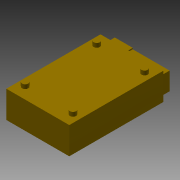
# Autodesk Inventor part: Vilros Pi Case
Saved by Autodesk Inventor 2015 SP1 (Build 190203100, 203)
## iProperties
Created: 2015-03-20
Part Number: Vilros Pi Case
Material: Generic
Document SubType Name: Modeling
Designer: steele
Density: 1 g/cm^3
Appearance: Gold
Author: steele
Autodesk Inventor part; units mm, degrees
ref_plane "YZ Plane" through (0, 0, 0) normal (1, 0, 0) x (0, 1, 0)
ref_plane "XZ Plane" through (0, 0, 0) normal (0, 1, 0) x (-1, 0, 0)
ref_plane "XY Plane" through (0, 0, 0) normal (0, 0, 1) x (1, 0, 0)
sketch "Sketch1" plane through (0, 0, 0) normal (0, 0, 1) x (1, 0, 0)
  line L0 (-30.75, -46) -> (30.75, -46)
  line L1 (30.75, -46) -> (30.75, 46)
  line L2 (30.75, 46) -> (-30.75, 46)
  line L3 (-30.75, 46) -> (-30.75, -46)
  line L4 (-30.75, -46) -> (30.75, 46) construction
  line L5 (30.75, -46) -> (-30.75, 46) construction
  point P0 (0, 0)
  dimension "d0" = 92
  dimension "d1" = 61.5
  constraints: 12 end point, 2 midpoint, 2 parallel, 1 horizontal, 1 perpendicular
  measures "d0" distance of L2.end L0.start
  measures "d1" distance of L0.start L0.end
extrude "Extrusion1" add sketch "Sketch1" along normal blind 26.4
sketch "Sketch3" plane through (0, 0, 26.4) normal (0, 0, 1) x (1, 0, 0)
  line L0 (-23.375, -34.95) -> (23.375, -34.95) construction
  line L1 (23.375, -34.95) -> (23.375, 34.95) construction
  line L2 (23.375, 34.95) -> (-23.375, 34.95) construction
  line L3 (-23.375, 34.95) -> (-23.375, -34.95) construction
  line L4 (-23.375, -34.95) -> (23.375, 34.95) construction
  line L5 (23.375, -34.95) -> (-23.375, 34.95) construction
  circle A0 centre (-23.375, -34.95) radius 3
  circle A1 centre (23.375, -34.95) radius 3
  circle A2 centre (23.375, 34.95) radius 3
  circle A3 centre (-23.375, 34.95) radius 3
  point P0 (0, 0)
  dimension "d5" = 46.75
  dimension "d6" = 69.9
  dimension "d7" = 6
  constraints: 12 end point, 4 centre point, 4 coincident, 3 equal radius, 2 midpoint, 2 parallel, 1 horizontal, 1 perpendicular
  measures "d5" distance of L1.end L2.end
  measures "d6" distance of L2.end L0.start
  measures "d7" diameter of A0
extrude "Extrusion2" add sketch "Sketch3" along normal blind 4
sketch "Sketch4" plane through (-30.75, 46, 0) normal (0, 1, 0) x (1, 0, 0)
  line L0 (0.1106, -5.25) -> (61.5, -5.25) construction
  line L1 (61.5, 0) -> (61.5, -26.4) construction
  line L2 (61.5, 0) -> (0, 0) construction
  line L3 (0, 0) -> (61.5, 0) construction
  line L4 (4, 0) -> (4, -26.4) construction
  line L5 (61.5, -26.4) -> (0, -26.4) construction
  line L6 (0, 0) -> (0, -26.4) construction
  line L7 (4, -5.25) -> (21.5, -5.25)
  line L8 (21.5, -5.25) -> (21.5, -20.75)
  line L9 (21.5, -20.75) -> (4, -20.75)
  line L10 (4, -20.75) -> (4, -5.25)
  point P0 (30.75, 0)
  dimension "d10" = 5.25
  dimension "d11" = 4
  dimension "d12" = 15.5
  dimension "d13" = 17.5
  constraints: 12 end point, 5 point on line, 2 horizontal, 2 parallel, 1 perpendicular, 1 vertical
  measures "d10" distance between parallel lines of L2 L0
  measures "d11" distance between parallel lines of L6 L4
  measures "d12" distance between parallel lines of L9 L0
  measures "d13" distance between parallel lines of L8 L4
extrude "Extrusion3" add sketch "Sketch4" along normal blind 10
sketch "Sketch5" plane through (-30.75, 46, 0) normal (0, 1, 0) x (1, 0, 0)
  line L0 (57.5, 0) -> (57.5, -26.4) construction
  line L1 (61.5, -26.4) -> (0, -26.4) construction
  line L2 (61.5, 0) -> (61.5, -26.4) construction
  line L3 (61.5, 0) -> (0, 0) construction
  line L4 (21.5, 0) -> (21.5, -26.4) construction
  line L5 (21.5, -2) -> (57.5, -2) construction
  line L6 (21.5, -5.25) -> (21.5, -20.75) construction
  line L7 (21.5, -19.5) -> (57.5, -19.5) construction
  line L8 (21.5, -2) -> (57.5, -2)
  line L9 (57.5, -2) -> (57.5, -19.5)
  line L10 (57.5, -19.5) -> (21.5, -19.5)
  line L11 (21.5, -19.5) -> (21.5, -2)
  point P0 (30.75, 0)
  dimension "d16" = 4
  dimension "d17" = 40
  dimension "d18" = 2
  dimension "d19" = 19.5
  constraints: 16 end point, 7 point on line, 2 horizontal, 2 parallel, 2 perpendicular, 2 vertical
  measures "d16" distance between parallel lines of L0 L2
  measures "d17" distance between parallel lines of L4 L2
  measures "d18" distance between parallel lines of L5 L3
  measures "d19" distance between parallel lines of L7 L3
extrude "Extrusion4" add sketch "Sketch5" along normal blind 10
body "Solid1"
